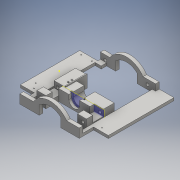
# Autodesk Inventor part: cutter carriage
Saved by Autodesk Inventor 2016 SP1 (Build 200210100, 210)
## iProperties
Created: 2017-04-28
Part Number: cutter carriage
Material: Generic
Document SubType Name: Modeling
Designer: Cole
Density: 1 g/cm^3
Appearance: Default
Author: Cole
Autodesk Inventor part; units mm, degrees
ref_plane "XZ Plane" through (0, 0, 0) normal (0, 1, 0) x (-1, 0, 0)
ref_plane "XY Plane" through (0, 0, 0) normal (0, 0, 1) x (1, 0, 0)
sketch "Sketch1" plane through (0, 0, 0) normal (0, 1, 0) x (-1, 0, 0)
  line L0 (-67, 0) -> (-67, -10)
  line L1 (0, -10) -> (0, 0)
  circle A0 centre (-10, -5) radius 1.6
  circle A1 centre (-57, -5) radius 1.6
  arc A2 (-15, 0) -> (-52, 0) centre (-33.5, -12.4452) ccw
  arc A3 (-21.4881, 0) -> (-45.5119, 0) centre (-33.5, -12.4452) ccw
  line L2 (0, 0) -> (-15, 0)
  line L3 (-52, 0) -> (-67, 0)
  line L4 (-21.4881, 0) -> (-21.4881, -10)
  line L5 (-45.5119, 0) -> (-45.5119, -10)
  line L6 (-67, -10) -> (-45.5119, -10)
  line L7 (-21.4881, -10) -> (0, -10)
  dimension "d0" = 3.2
  dimension "d1" = 67
  dimension "d2" = 10
  dimension "d3" = 3.2
  dimension "d4" = 47
  dimension "d5" = 10
  dimension "d13" = 5
  dimension "d14" = 5
  dimension "d15" = 5
  dimension "d16" = 10
  constraints: 16 end point, 5 parallel, 4 centre point, 4 point on circle, 2 horizontal, 2 perpendicular, 1 coincident
  measures "d0" diameter of A0
  measures "d1" distance of L0.end L1.start
  measures "d2" distance of L1.start L1.end
  measures "d3" diameter of A1
  measures "d4" distance of A1.centre A0.centre
  measures "d5" distance from line of L1 A0.centre
  measures "d13" horizontal distance of L2.end A0.centre
  measures "d14" horizontal distance of A1.centre L3.start
  measures "d15" radial gap between concentric circles of A2 A3
  measures "d16" distance of L4.start L4.end
extrude "Extrusion3" add sketch "Sketch1" along normal blind 3
sketch "Sketch3" plane through (0, 0, 0) normal (0, -1, 0) x (1, 0, 0)
  circle A0 centre (57, -5) radius 1.6 projected
  circle A1 centre (10, -5) radius 1.6 projected
  line L0 (0, 0) -> (0, -10) projected
  line L1 (0, -10) -> (21.4881, -10) projected
  line L2 (21.4881, -10) -> (21.4881, 0) projected
  arc A2 (45.5119, 0) -> (21.4881, 0) centre (33.5, -12.4452) ccw projected
  line L3 (45.5119, 0) -> (45.5119, -10) projected
  line L4 (45.5119, -10) -> (67, -10) projected
  line L5 (67, -10) -> (67, 0) projected
  line L6 (67, 0) -> (52, 0) projected
  arc A3 (52, 0) -> (15, 0) centre (33.5, -12.4452) ccw projected
  line L7 (15, 0) -> (0, 0) projected
extrude "Extrusion4" add sketch "Sketch3" along normal blind 1 contours A0 | A1 | L7 A3 L6 L5 L4 L3 A2 L2 L1 L0
ref_plane "Work Plane1" through (10, 87, -5) normal (0, 1, 0) x (1, 0, 0)
sketch "Sketch4" plane through (10, 87, -5) normal (0, 1, 0) x (1, 0, 0)
  line L0 (-10, -5) -> (-10, 5) projected
  line L1 (-10, 5) -> (11.4881, 5) projected
  line L2 (11.4881, 5) -> (11.4881, -5) projected
  arc A0 (11.4881, -5) -> (35.5119, -5) centre (23.5, 7.4452) ccw projected
  line L3 (35.5119, -5) -> (35.5119, 5) projected
  line L4 (35.5119, 5) -> (57, 5) projected
  line L5 (57, 5) -> (57, -5) projected
  line L6 (57, -5) -> (42, -5) projected
  arc A1 (5, -5) -> (42, -5) centre (23.5, 7.4452) ccw projected
  line L7 (5, -5) -> (-10, -5) projected
extrude "Extrusion5" add sketch "Sketch4" along normal blind 1
sketch "Sketch5" plane through (10, 87, -5) normal (0, -1, 0) x (1, 0, 0)
  circle A0 centre (0, 0) radius 1.6 projected
  circle A1 centre (47, 0) radius 1.6 projected
  line L0 (-10, 5) -> (-10, -5) projected
  line L1 (-10, -5) -> (11.4881, -5) projected
  line L2 (11.4881, -5) -> (11.4881, 5) projected
  arc A2 (35.5119, 5) -> (11.4881, 5) centre (23.5, -7.4452) ccw projected
  line L3 (35.5119, 5) -> (35.5119, -5) projected
  line L4 (35.5119, -5) -> (57, -5) projected
  line L5 (57, -5) -> (57, 5) projected
  line L6 (57, 5) -> (42, 5) projected
  arc A3 (42, 5) -> (5, 5) centre (23.5, -7.4452) ccw projected
  line L7 (5, 5) -> (-10, 5) projected
extrude "Extrusion6" add sketch "Sketch5" along normal blind 3
sketch "Sketch7" plane through (21.4881, 3, -10) normal (0, 0, -1) x (-1, 0, 0)
  line L0 (13.0881, -3) -> (13.0881, 0) projected
  line L1 (16.8881, -4) -> (36.8881, -4)
  line L2 (36.8881, -4) -> (36.8881, 85)
  line L3 (36.8881, 85) -> (16.8881, 85)
  line L4 (16.8881, 85) -> (16.8881, -4)
  line L5 (0, 85) -> (21.4881, 85) projected
  point P0 (21.4881, -3)
  dimension "d27" = 3.8
  dimension "d28" = 20
  constraints: 8 end point, 2 parallel, 1 collinear, 1 horizontal, 1 perpendicular
  measures "d27" distance between parallel lines of L4 L0
  measures "d28" distance of L1.start L1.end
extrude "Extrusion7" add sketch "Sketch7" against normal blind 3
sketch "Sketch8" plane through (21.4881, 3, -7) normal (0, 0, 1) x (1, 0, 0)
  line L0 (-21.4881, -4) -> (-36.9881, -4)
  line L1 (-36.9881, -4) -> (-36.9881, 12)
  line L2 (-36.9881, 12) -> (-21.4881, 12)
  line L3 (-21.4881, 12) -> (-21.4881, -4)
  line L4 (-21.4881, -4) -> (-21.4881, 0) projected
  point P0 (-21.4881, -3)
  dimension "d31" = 16
  constraints: 8 end point, 2 parallel, 1 collinear, 1 horizontal, 1 perpendicular
  measures "d31" distance of L0.end L1.end
extrude "Extrusion8" cut sketch "Sketch8" against normal through all
sketch "Sketch9" plane through (52, 88, 0) normal (0, 0, 1) x (1, 0, 0)
  line L0 (14, 5.5795) -> (24.4678, 5.5795)
  line L1 (24.4678, 5.5795) -> (24.4678, -94.3099)
  line L2 (24.4678, -94.3099) -> (14, -94.3099)
  line L3 (14, -94.3099) -> (14, 5.5795)
  line L4 (15, 0) -> (15, -4) projected
  point P0 (-52, -88)
  dimension "d34" = 1
  constraints: 8 end point, 2 parallel, 1 horizontal, 1 perpendicular
  measures "d34" distance from line of L4 L0.start
extrude "Extrusion9" cut sketch "Sketch9" against normal through all
ref_plane "Work Plane2" through (33.5, 88, -12.4452) normal (1, 0, 0) x (0, 1, 0)
mirror "Mirror1" about plane through (33.5, 88, -12.4452) normal (1, 0, 0) of "Extrusion7"
sketch "Sketch10" plane through (66, -1, -7) normal (0, 0, 1) x (1, 0, 0)
  line L0 (16.4, 0) -> (0, 0)
  line L1 (0, 0) -> (0, 16)
  line L2 (0, 16) -> (16.4, 16)
  line L3 (16.4, 16) -> (16.4, 0)
  point P0 (-66, 1)
  constraints: 8 end point, 2 parallel, 1 horizontal, 1 perpendicular
extrude "Extrusion10" cut sketch "Sketch10" against normal through all
sketch "Sketch11" plane through (10, 87, -5) normal (0, -1, 0) x (1, 0, 0)
  circle A0 centre (0, 0) radius 1.6 projected
  circle A1 centre (47, 0) radius 1.6 projected
  point P0 (-10, 5)
extrude "Extrusion11" cut sketch "Sketch11" against normal through all
sketch "Sketch12" plane through (21.4881, 3, -7) normal (0, 0, 1) x (1, 0, 0)
  line L0 (-43.9155, 94.6628) -> (-16.8881, 94.6628)
  line L1 (-16.8881, 94.6628) -> (-16.8881, 78)
  line L2 (-16.8881, 78) -> (-43.9155, 78)
  line L3 (-43.9155, 78) -> (-43.9155, 94.6628)
  line L4 (-21.4881, 85) -> (-36.8881, 85) projected
  point P0 (-21.4881, -3)
  dimension "d42" = 7
  constraints: 8 end point, 2 parallel, 1 horizontal, 1 perpendicular
  measures "d42" distance between parallel lines of L2 L4
extrude "Extrusion12" cut sketch "Sketch12" along normal through all both and the other way through all
sketch "Sketch13" plane through (10, 84, -5) normal (0, -1, 0) x (1, 0, 0)
  line L0 (-5.4, -2) -> (1.4367, -2)
  line L1 (1.4367, -2) -> (1.4367, -5)
  line L2 (1.4367, -5) -> (-5.4, -5)
  line L3 (-5.4, -5) -> (-5.4, -2)
  line L4 (-5.4, -5) -> (-5.4, 5) projected
  point P0 (-10, 5)
  constraints: 8 end point, 2 parallel, 1 collinear, 1 horizontal, 1 perpendicular
extrude "Extrusion13" add sketch "Sketch13" along normal blind 6
sketch "Sketch14" plane through (45.5119, -1, -10) normal (0, 0, -1) x (-1, 0, 0)
  circle A0 centre (-25.8881, 20) radius 0.5
  line L0 (-36.8881, 16) -> (-36.8881, 89) projected
  line L1 (-36.8881, 16) -> (-20.4881, 16) projected
  circle A1 centre (49.9119, 20) radius 0.5
  line L2 (45.5119, 16) -> (60.9119, 16) projected
  line L3 (60.9119, 16) -> (60.9119, 82) projected
  point P0 (45.5119, 1)
  dimension "d47" = 1
  dimension "d48" = 11
  dimension "d49" = 4
  dimension "d50" = 1
  dimension "d51" = 4
  dimension "d52" = 11
  constraints: 2 centre point
  measures "d47" diameter of A0
  measures "d48" distance from line of L0 A0.centre
  measures "d49" distance from line of L1 A0.centre
  measures "d50" diameter of A1
  measures "d51" distance from line of L2 A1.centre
  measures "d52" distance from line of A1.centre L3
extrude "Extrusion14" cut sketch "Sketch14" against normal blind 6
ref_plane "Work Plane3" through (0, 31, 0) normal (0, 1, 0) x (1, 0, 0)
sketch "Sketch15" plane through (0, 31, 0) normal (0, 1, 0) x (1, 0, 0)
  circle A0 centre (10, 5) radius 1.6 projected
  circle A1 centre (57, 5) radius 1.6 projected
  circle A2 centre (10, 5) radius 1.6
  circle A3 centre (57, 5) radius 1.6
  line L0 (6, 10) -> (61, 10)
  line L1 (61, 10) -> (61, 0.35)
  line L2 (61, 0.35) -> (6, 0.35)
  line L3 (6, 0.35) -> (6, 10)
  point P0 (0, 0)
  dimension "d56" = 3.2
  dimension "d57" = 3.2
  dimension "d58" = 4
  dimension "d59" = 4.65
  dimension "d60" = 4
  dimension "d61" = 5
  constraints: 8 end point, 2 centre point, 2 parallel, 1 horizontal, 1 perpendicular
  measures "d56" diameter of A2
  measures "d57" diameter of A3
  measures "d58" distance from line of L3 A0.centre
  measures "d59" distance from line of A0.centre L2
  measures "d60" distance from line of L1 A1.centre
  measures "d61" distance from line of L0 A0.centre
extrude "Extrusion15" add sketch "Sketch15" along normal blind 12
sketch "Sketch16" plane through (6, 31, -0.35) normal (0, 0, 1) x (1, 0, 0)
  line L0 (2.4, 0) -> (2.4, 12) projected
  circle A0 centre (9.4, 6.5) radius 0.9
  line L1 (0, 12) -> (55, 12) projected
  circle A1 centre (9.4, 10.5) radius 0.85
  point P0 (-6, -31)
  dimension "d64" = 7
  dimension "d65" = 1.8
  dimension "d66" = 5.5
  dimension "d67" = 1.7
  dimension "d69" = 4
  constraints: 2 centre point
  measures "d64" distance from line of L0 A0.centre
  measures "d65" diameter of A0
  measures "d66" distance from line of L1 A0.centre
  measures "d67" diameter of A1
  measures "d69" distance of A1.centre A0.centre
extrude "Extrusion16" cut sketch "Sketch16" against normal blind 7
sketch "Sketch17" plane through (0, 31, 0) normal (0, -1, 0) x (1, 0, 0)
  line L0 (6, -0.35) -> (16, -0.35)
  line L1 (16, -0.35) -> (16, -10)
  line L2 (16, -10) -> (6, -10)
  line L3 (6, -10) -> (6, -0.35)
  circle A0 centre (10, -5) radius 1.6 projected
  line L4 (33.5, -0.35) -> (33.5, -7.7641)
  line L5 (61, -0.35) -> (51, -0.35)
  line L6 (51, -0.35) -> (51, -10)
  line L7 (51, -10) -> (61, -10)
  line L8 (61, -10) -> (61, -0.35)
  circle A1 centre (57, -5) radius 1.6
  point P0 (0, 0)
  dimension "d75" = 10
  constraints: 18 end point, 5 symmetric about line, 2 parallel, 1 centre point, 1 horizontal, 1 perpendicular, 1 other
  measures "d75" distance of L1.end L2.end
extrude "Extrusion17" add sketch "Sketch17" along normal blind 19
sketch "Sketch18" plane through (0, 43, 0) normal (0, 1, 0) x (1, 0, 0)
  point P0 (0, 0)
sketch "Sketch19" plane through (0, 43, 0) normal (0, 1, 0) x (1, 0, 0)
  circle A0 centre (10, 5) radius 1.6 projected
  line L0 (16, 0.35) -> (6, 0.35) projected
  line L1 (6, 0.35) -> (6, 10) projected
  line L2 (6, 10) -> (16, 10) projected
  line L3 (16, 10) -> (16, 0.35) projected
  point P0 (0, 0)
extrude "Extrusion18" add sketch "Sketch19" along normal blind 12
sketch "Sketch20" plane through (16, 43, -0.35) normal (1, 0, 0) x (0, 0, -1)
  line L0 (9.65, 0) -> (0, 0) projected
  line L1 (9.65, 0) -> (9.65, 12) projected
  line L2 (0, 12) -> (9.65, 12) projected
  line L3 (0, 0) -> (0, 12) projected
  point P0 (-0.35, -43)
extrude "Extrusion19" add sketch "Sketch20" along normal blind 3
sketch "Sketch21" plane through (16, 31, -0.35) normal (0, 0, 1) x (1, 0, 0)
  line L0 (3, 12) -> (2, 12)
  line L1 (2, 12) -> (2, 24)
  line L2 (2, 24) -> (3, 24)
  line L3 (3, 24) -> (3, 12)
  line L4 (3, 12) -> (45, 12) projected
  line L5 (3, 24) -> (3, 12) projected
  point P0 (-16, -31)
  dimension "d82" = 1
  constraints: 8 end point, 2 collinear, 2 parallel, 1 horizontal, 1 perpendicular
  measures "d82" distance of L1.end L2.end
extrude "Extrusion20" add sketch "Sketch21" along normal blind 1
sketch "Sketch22" plane through (18, 43, -0.35) normal (0, -1, 0) x (1, 0, 0)
  line L0 (1, 0) -> (0, 0) projected
  line L1 (1, 0) -> (1, 1) projected
  line L2 (0, 1) -> (1, 1) projected
  line L3 (0, 0) -> (0, 1) projected
  point P0 (-18, 0.35)
extrude "Extrusion21" add sketch "Sketch22" along normal up to surface (12 mm away)
sketch "Sketch24" plane through (6, 12, -0.35) normal (0, 0, 1) x (1, 0, 0)
  line L0 (-0.5579, 19) -> (55.8525, 19)
  line L1 (55.8525, 19) -> (55.8525, 7)
  line L2 (55.8525, 7) -> (-0.5579, 7)
  line L3 (-0.5579, 7) -> (-0.5579, 19)
  line L4 (55, 0) -> (45, 0) projected
  point P0 (-6, -12)
  dimension "d88" = 7
  constraints: 8 end point, 2 parallel, 1 horizontal, 1 perpendicular
  measures "d88" distance between parallel lines of L4 L2
extrude "Extrusion22" cut sketch "Sketch24" against normal blind 7
sketch "Sketch25" plane through (21.4881, 3, -7) normal (0, 0, 1) x (1, 0, 0)
  circle A0 centre (-31.8881, 74.5) radius 0.5
  line L0 (-16.8881, 78) -> (-36.8881, 78) projected
  line L1 (-36.8881, 78) -> (-36.8881, 12) projected
  circle A1 centre (-19.8881, 74.5) radius 0.5
  circle A2 centre (-29.8881, 22) radius 0.5
  line L2 (-36.8881, 12) -> (-21.4881, 12) projected
  point P0 (-21.4881, -3)
  dimension "d91" = 3.5
  dimension "d92" = 5
  dimension "d93" = 17
  dimension "d94" = 3.5
  dimension "d95" = 1
  dimension "d96" = 1
  dimension "d97" = 7
  dimension "d98" = 10
  dimension "d99" = 1
  constraints: 3 centre point
  measures "d91" distance from line of L0 A0.centre
  measures "d92" distance from line of L1 A0.centre
  measures "d93" distance from line of L1 A1.centre
  measures "d94" distance from line of L0 A1.centre
  measures "d95" diameter of A0
  measures "d96" diameter of A1
  measures "d97" distance from line of L1 A2.centre
  measures "d98" distance from line of L2 A2.centre
  measures "d99" diameter of A2
extrude "Extrusion23" cut sketch "Sketch25" against normal through all
sketch "Sketch26" plane through (0, 0, 0) normal (0, 1, 0) x (-1, 0, 0)
  circle A0 centre (-33.4999, -5) radius 6
  line L0 (-45.5119, 0) -> (-45.5119, -10) projected
  line L1 (-21.4881, -10) -> (0, -10) projected
  point P0 (0, 0)
  dimension "d102" = 12
  dimension "d103" = 12.012
  dimension "d104" = 5
  constraints: 1 centre point
  measures "d102" diameter of A0
  measures "d103" distance from line of L0 A0.centre
  measures "d104" distance from line of L1 A0.centre
extrude "Extrusion24" add sketch "Sketch26" along normal blind 50 separate body
sketch "Sketch27" plane through (51, 31, -10) normal (0, 0, -1) x (-1, 0, 0)
  line L0 (45, -19) -> (45, 24) projected
  line L1 (45, 24) -> (32, 24) projected
  line L2 (32, 12) -> (32, 24) projected
  line L3 (-10, 12) -> (32, 12) projected
  line L4 (-10, 12) -> (-10, -19) projected
  line L5 (0, -19) -> (-10, -19) projected
  line L6 (0, 0) -> (0, -19) projected
  line L7 (35, 0) -> (0, 0) projected
  line L8 (35, 0) -> (35, -19) projected
  line L9 (45, -19) -> (35, -19) projected
  point P0 (51, -31)
extrude "Extrusion25" add sketch "Sketch27" along normal blind 3 bodies 1
sketch "Sketch28" plane through (61, 31, -0.35) normal (0, 0, 1) x (1, 0, 0)
  line L0 (-21.5001, -31) -> (-21.5001, 19) projected
  line L1 (-33.5001, -31) -> (-33.5001, 19) projected
  line L2 (-33.5001, 12) -> (-21.5001, 12)
  line L3 (-21.5001, 12) -> (-21.5001, 0)
  line L4 (-21.5001, 0) -> (-33.5001, 0)
  line L5 (-33.5001, 0) -> (-33.5001, 12)
  point P0 (-61, -31)
  constraints: 8 end point, 2 parallel, 1 horizontal, 1 perpendicular
extrude "Extrusion26" cut sketch "Sketch28" against normal blind 5 bodies 1
sketch "Sketch29" plane through (33.4999, 50, -5) normal (0, 1, 0) x (1, 0, 0)
  circle A0 centre (0, 0) radius 6 projected
  point P0 (-33.4999, -5)
extrude "Extrusion27" cut sketch "Sketch29" against normal through all bodies 1
ref_plane "Work Plane5" through (0, 30, 0) normal (0, 1, 0) x (1, 0, 0)
sketch "Sketch31" plane through (0, 31, 0) normal (0, -1, 0) x (1, 0, 0)
  arc A0 (27.5101, -5.35) -> (39.4897, -5.35) centre (33.4999, -5) ccw
  line L0 (27.5101, -5.35) -> (27.4999, -5.35)
  line L1 (27.4999, -5.35) -> (27.4999, -0.35)
  line L2 (27.4999, -0.35) -> (19, -0.35)
  line L3 (18, -0.35) -> (16, -0.35)
  line L4 (16, -7.35) -> (16, -13)
  line L5 (51, -13) -> (16, -13)
  line L6 (51, -13) -> (51, -7.35)
  line L7 (51, -0.35) -> (39.4999, -0.35)
  line L8 (39.4999, -0.35) -> (39.4999, -5.35)
  line L9 (39.4999, -5.35) -> (39.4897, -5.35)
  line L10 (16, -7.35) -> (16, -0.35)
  line L11 (51, -7.35) -> (51, -0.35)
  line L12 (18, -0.35) -> (19, -0.35)
  point P0 (0, 0)
  constraints: 26 end point, 2 centre point, 2 point on circle
extrude "Extrusion29" add sketch "Sketch31" along normal blind 5 bodies 1
sketch "Sketch30" plane through (0, 30, 0) normal (0, 1, 0) x (1, 0, 0)
  arc A0 (41.4999, 5) -> (25.4999, 5) centre (33.4999, 5) ccw
  arc A1 (39.4897, 5.35) -> (27.5101, 5.35) centre (33.4999, 5) ccw
  line L0 (41.4999, 5) -> (41.4999, -3)
  line L1 (41.4999, -3) -> (25.4999, -3)
  line L2 (25.4999, -3) -> (25.4999, 5)
  point P0 (0, 0)
  dimension "d114" = 16
  constraints: 6 end point, 4 point on circle, 3 tangent, 2 centre point, 1 concentric, 1 parallel
  measures "d114" diameter of A0
extrude "Extrusion28" cut sketch "Sketch30" along normal mid plane 2.2 bodies 1
body "Solid2"
body "Solid3"
